Autodesk Fusion 360 part; units mm, degrees
(part 2 of 7)
  spline S15 degree 5 poles (6.7493, -2.5075) (6.7469, -2.5043) (6.7422, -2.4978) (6.7351, -2.4882) (6.7256, -2.4755) (6.7136, -2.4596) (6.7016, -2.4438) (6.6895, -2.4282) (6.6774, -2.4126) (6.6652, -2.3971) (6.653, -2.3817) (6.6407, -2.3664) (6.6283, -2.3512) (6.6159, -2.336) (6.6034, -2.321) (6.5909, -2.3061) (6.5783, -2.2913) (6.5657, -2.2766) (6.553, -2.2619) (6.5402, -2.2474) (6.5274, -2.233) (6.5145, -2.2186) (6.5016, -2.2044) (6.4886, -2.1903) (6.4756, -2.1763) (6.4625, -2.1624) (6.4493, -2.1486) (6.4361, -2.1349) (6.4229, -2.1213) (6.4095, -2.1078) (6.3962, -2.0944) (6.3827, -2.0812) (6.3692, -2.068) (6.3557, -2.055) (6.3421, -2.0421) (6.3284, -2.0293) (6.3147, -2.0166) (6.301, -2.004) (6.2871, -1.9916) (6.2733, -1.9792) (6.2593, -1.967) (6.2453, -1.955) (6.2313, -1.943) (6.2172, -1.9312) (6.203, -1.9195) (6.1888, -1.9079) (6.1745, -1.8965) (6.1602, -1.8852) (6.1458, -1.874) (6.1313, -1.863) (6.1168, -1.8521) (6.1023, -1.8414) (6.0876, -1.8308) (6.0729, -1.8204) (6.0582, -1.8101) (6.0434, -1.8) (6.0285, -1.79) (6.0136, -1.7802) (5.9986, -1.7705) (5.9836, -1.761) (5.9685, -1.7518) (5.9533, -1.7427) (5.938, -1.7339) (5.9226, -1.7254) (5.9071, -1.717) (5.8916, -1.7089) (5.8761, -1.7008) (5.8605, -1.6929) (5.8448, -1.6852) (5.8291, -1.6778) (5.8132, -1.671) (5.8002, -1.6661) (5.7904, -1.6628) (5.7838, -1.6608) (5.7805, -1.6598) knots -1 -1 -1 -1 -1 -1 -0.98571429 -0.97142857 -0.95714286 -0.94285714 -0.92857143 -0.91428571 -0.9 -0.88571429 -0.87142857 -0.85714286 -0.84285714 -0.82857143 -0.81428571 -0.8 -0.78571429 -0.77142857 -0.75714286 -0.74285714 -0.72857143 -0.71428571 -0.7 -0.68571429 -0.67142857 -0.65714286 -0.64285714 -0.62857143 -0.61428571 -0.6 -0.58571429 -0.57142857 -0.55714286 -0.54285714 -0.52857143 -0.51428571 -0.5 -0.48571429 -0.47142857 -0.45714286 -0.44285714 -0.42857143 -0.41428571 -0.4 -0.38571429 -0.37142857 -0.35714286 -0.34285714 -0.32857143 -0.31428571 -0.3 -0.28571429 -0.27142857 -0.25714286 -0.24285714 -0.22857143 -0.21428571 -0.2 -0.18571429 -0.17142857 -0.15714286 -0.14285714 -0.12857143 -0.11428571 -0.1 -0.08571429 -0.07142857 -0.05714286 -0.04285714 -0.02857143 -0.01428571 0 0 0 0 0 0
  line L15 (5.7805, -1.6598) -> (5.4506, -1.5651)
  arc A31 (5.3118, -1.3245) -> (5.4506, -1.5651) centre (5.5058, -1.3729) ccw
  arc A32 (5.3118, -1.3245) -> (5.4143, -0.8091) centre (0, 0) ccw
  arc A33 (5.6347, -0.6399) -> (5.4143, -0.8091) centre (5.6121, -0.8386) ccw
  line L16 (5.6347, -0.6399) -> (5.9756, -0.6786)
  spline S16 degree 5 poles (5.9756, -0.6786) (5.9791, -0.679) (5.9859, -0.6797) (5.9963, -0.6804) (6.0101, -0.6808) (6.0275, -0.6806) (6.0448, -0.6798) (6.0622, -0.6786) (6.0796, -0.6773) (6.0971, -0.6758) (6.1145, -0.6742) (6.132, -0.6724) (6.1495, -0.6704) (6.167, -0.6682) (6.1845, -0.6656) (6.202, -0.6628) (6.2196, -0.6598) (6.2371, -0.6566) (6.2546, -0.6532) (6.2722, -0.6497) (6.2897, -0.646) (6.3073, -0.6422) (6.3249, -0.6382) (6.3424, -0.634) (6.36, -0.6297) (6.3776, -0.6252) (6.3951, -0.6205) (6.4127, -0.6157) (6.4303, -0.6108) (6.4478, -0.6057) (6.4654, -0.6004) (6.4829, -0.595) (6.5005, -0.5895) (6.5181, -0.5838) (6.5356, -0.578) (6.5532, -0.5721) (6.5707, -0.566) (6.5882, -0.5598) (6.6058, -0.5535) (6.6233, -0.547) (6.6408, -0.5404) (6.6583, -0.5336) (6.6758, -0.5268) (6.6933, -0.5198) (6.7108, -0.5127) (6.7283, -0.5055) (6.7457, -0.4981) (6.7632, -0.4906) (6.7806, -0.483) (6.7981, -0.4753) (6.8155, -0.4675) (6.8329, -0.4595) (6.8503, -0.4514) (6.8677, -0.4432) (6.8851, -0.4349) (6.9024, -0.4265) (6.9198, -0.418) (6.9371, -0.4093) (6.9544, -0.4006) (6.9717, -0.3917) (6.989, -0.3827) (7.0063, -0.3736) (7.0235, -0.3644) (7.0408, -0.355) (7.058, -0.3456) (7.0752, -0.3361) (7.0924, -0.3264) (7.1095, -0.3167) (7.1267, -0.3068) (7.1438, -0.2968) (7.1609, -0.2867) (7.1746, -0.2786) (7.1848, -0.2724) (7.1917, -0.2683) (7.1951, -0.2662) knots 0 0 0 0 0 0 0.01428571 0.02857143 0.04285714 0.05714286 0.07142857 0.08571429 0.1 0.11428571 0.12857143 0.14285714 0.15714286 0.17142857 0.18571429 0.2 0.21428571 0.22857143 0.24285714 0.25714286 0.27142857 0.28571429 0.3 0.31428571 0.32857143 0.34285714 0.35714286 0.37142857 0.38571429 0.4 0.41428571 0.42857143 0.44285714 0.45714286 0.47142857 0.48571429 0.5 0.51428571 0.52857143 0.54285714 0.55714286 0.57142857 0.58571429 0.6 0.61428571 0.62857143 0.64285714 0.65714286 0.67142857 0.68571429 0.7 0.71428571 0.72857143 0.74285714 0.75714286 0.77142857 0.78571429 0.8 0.81428571 0.82857143 0.84285714 0.85714286 0.87142857 0.88571429 0.9 0.91428571 0.92857143 0.94285714 0.95714286 0.97142857 0.98571429 1 1 1 1 1 1
  arc A34 (7.1951, -0.2662) -> (7.1951, 0.2662) centre (0, 0) ccw
  spline S17 degree 5 poles (7.1951, 0.2662) (7.1917, 0.2683) (7.1848, 0.2724) (7.1746, 0.2786) (7.1609, 0.2867) (7.1438, 0.2968) (7.1267, 0.3068) (7.1095, 0.3167) (7.0924, 0.3264) (7.0752, 0.3361) (7.058, 0.3456) (7.0408, 0.355) (7.0235, 0.3644) (7.0063, 0.3736) (6.989, 0.3827) (6.9717, 0.3917) (6.9544, 0.4006) (6.9371, 0.4093) (6.9198, 0.418) (6.9024, 0.4265) (6.8851, 0.4349) (6.8677, 0.4432) (6.8503, 0.4514) (6.8329, 0.4595) (6.8155, 0.4675) (6.7981, 0.4753) (6.7806, 0.483) (6.7632, 0.4906) (6.7457, 0.4981) (6.7283, 0.5055) (6.7108, 0.5127) (6.6933, 0.5198) (6.6758, 0.5268) (6.6583, 0.5336) (6.6408, 0.5404) (6.6233, 0.547) (6.6058, 0.5535) (6.5882, 0.5598) (6.5707, 0.566) (6.5532, 0.5721) (6.5356, 0.578) (6.5181, 0.5838) (6.5005, 0.5895) (6.4829, 0.595) (6.4654, 0.6004) (6.4478, 0.6057) (6.4303, 0.6108) (6.4127, 0.6157) (6.3951, 0.6205) (6.3776, 0.6252) (6.36, 0.6297) (6.3424, 0.634) (6.3249, 0.6382) (6.3073, 0.6422) (6.2897, 0.646) (6.2722, 0.6497) (6.2546, 0.6532) (6.2371, 0.6566) (6.2196, 0.6598) (6.202, 0.6628) (6.1845, 0.6656) (6.167, 0.6682) (6.1495, 0.6704) (6.132, 0.6724) (6.1145, 0.6742) (6.0971, 0.6758) (6.0796, 0.6773) (6.0622, 0.6786) (6.0448, 0.6798) (6.0275, 0.6806) (6.0101, 0.6808) (5.9963, 0.6804) (5.9859, 0.6797) (5.9791, 0.679) (5.9756, 0.6786) knots -1 -1 -1 -1 -1 -1 -0.98571429 -0.97142857 -0.95714286 -0.94285714 -0.92857143 -0.91428571 -0.9 -0.88571429 -0.87142857 -0.85714286 -0.84285714 -0.82857143 -0.81428571 -0.8 -0.78571429 -0.77142857 -0.75714286 -0.74285714 -0.72857143 -0.71428571 -0.7 -0.68571429 -0.67142857 -0.65714286 -0.64285714 -0.62857143 -0.61428571 -0.6 -0.58571429 -0.57142857 -0.55714286 -0.54285714 -0.52857143 -0.51428571 -0.5 -0.48571429 -0.47142857 -0.45714286 -0.44285714 -0.42857143 -0.41428571 -0.4 -0.38571429 -0.37142857 -0.35714286 -0.34285714 -0.32857143 -0.31428571 -0.3 -0.28571429 -0.27142857 -0.25714286 -0.24285714 -0.22857143 -0.21428571 -0.2 -0.18571429 -0.17142857 -0.15714286 -0.14285714 -0.12857143 -0.11428571 -0.1 -0.08571429 -0.07142857 -0.05714286 -0.04285714 -0.02857143 -0.01428571 0 0 0 0 0 0
  line L17 (5.9756, 0.6786) -> (5.6347, 0.6399)
  arc A35 (5.4143, 0.8091) -> (5.6347, 0.6399) centre (5.6121, 0.8386) ccw
  arc A36 (5.4143, 0.8091) -> (5.3118, 1.3245) centre (0, 0) ccw
  arc A37 (5.4506, 1.5651) -> (5.3118, 1.3245) centre (5.5058, 1.3729) ccw
  line L18 (5.4506, 1.5651) -> (5.7805, 1.6598)
  spline S18 degree 5 poles (5.7805, 1.6598) (5.7838, 1.6608) (5.7904, 1.6628) (5.8002, 1.6661) (5.8132, 1.671) (5.8291, 1.6778) (5.8448, 1.6852) (5.8605, 1.6929) (5.8761, 1.7008) (5.8916, 1.7089) (5.9071, 1.717) (5.9226, 1.7254) (5.938, 1.7339) (5.9533, 1.7427) (5.9685, 1.7518) (5.9836, 1.761) (5.9986, 1.7705) (6.0136, 1.7802) (6.0285, 1.79) (6.0434, 1.8) (6.0582, 1.8101) (6.0729, 1.8204) (6.0876, 1.8308) (6.1023, 1.8414) (6.1168, 1.8521) (6.1313, 1.863) (6.1458, 1.874) (6.1602, 1.8852) (6.1745, 1.8965) (6.1888, 1.9079) (6.203, 1.9195) (6.2172, 1.9312) (6.2313, 1.943) (6.2453, 1.955) (6.2593, 1.967) (6.2733, 1.9792) (6.2871, 1.9916) (6.301, 2.004) (6.3147, 2.0166) (6.3284, 2.0293) (6.3421, 2.0421) (6.3557, 2.055) (6.3692, 2.068) (6.3827, 2.0812) (6.3962, 2.0944) (6.4095, 2.1078) (6.4229, 2.1213) (6.4361, 2.1349) (6.4493, 2.1486) (6.4625, 2.1624) (6.4756, 2.1763) (6.4886, 2.1903) (6.5016, 2.2044) (6.5145, 2.2186) (6.5274, 2.233) (6.5402, 2.2474) (6.553, 2.2619) (6.5657, 2.2766) (6.5783, 2.2913) (6.5909, 2.3061) (6.6034, 2.321) (6.6159, 2.336) (6.6283, 2.3512) (6.6407, 2.3664) (6.653, 2.3817) (6.6652, 2.3971) (6.6774, 2.4126) (6.6895, 2.4282) (6.7016, 2.4438) (6.7136, 2.4596) (6.7256, 2.4755) (6.7351, 2.4882) (6.7422, 2.4978) (6.7469, 2.5043) (6.7493, 2.5075) knots 0 0 0 0 0 0 0.01428571 0.02857143 0.04285714 0.05714286 0.07142857 0.08571429 0.1 0.11428571 0.12857143 0.14285714 0.15714286 0.17142857 0.18571429 0.2 0.21428571 0.22857143 0.24285714 0.25714286 0.27142857 0.28571429 0.3 0.31428571 0.32857143 0.34285714 0.35714286 0.37142857 0.38571429 0.4 0.41428571 0.42857143 0.44285714 0.45714286 0.47142857 0.48571429 0.5 0.51428571 0.52857143 0.54285714 0.55714286 0.57142857 0.58571429 0.6 0.61428571 0.62857143 0.64285714 0.65714286 0.67142857 0.68571429 0.7 0.71428571 0.72857143 0.74285714 0.75714286 0.77142857 0.78571429 0.8 0.81428571 0.82857143 0.84285714 0.85714286 0.87142857 0.88571429 0.9 0.91428571 0.92857143 0.94285714 0.95714286 0.97142857 0.98571429 1 1 1 1 1 1
  arc A38 (6.7493, 2.5075) -> (6.5455, 2.9994) centre (0, 0) ccw
  spline S19 degree 5 poles (6.5455, 2.9994) (6.5416, 3) (6.5337, 3.0012) (6.5219, 3.003) (6.5061, 3.0053) (6.4864, 3.008) (6.4668, 3.0107) (6.4472, 3.0133) (6.4276, 3.0157) (6.408, 3.018) (6.3885, 3.0203) (6.3689, 3.0224) (6.3495, 3.0244) (6.33, 3.0263) (6.3105, 3.0281) (6.2911, 3.0298) (6.2718, 3.0314) (6.2524, 3.0329) (6.2331, 3.0342) (6.2138, 3.0355) (6.1945, 3.0366) (6.1753, 3.0377) (6.1561, 3.0386) (6.1369, 3.0394) (6.1178, 3.0401) (6.0987, 3.0406) (6.0796, 3.0411) (6.0606, 3.0414) (6.0416, 3.0417) (6.0227, 3.0418) (6.0038, 3.0418) (5.9849, 3.0417) (5.9661, 3.0414) (5.9473, 3.0411) (5.9285, 3.0406) (5.9098, 3.04) (5.8911, 3.0392) (5.8725, 3.0384) (5.8539, 3.0374) (5.8354, 3.0363) (5.8169, 3.0351) (5.7985, 3.0338) (5.7801, 3.0323) (5.7618, 3.0307) (5.7435, 3.0289) (5.7252, 3.027) (5.7071, 3.025) (5.6889, 3.0229) (5.6709, 3.0206) (5.6528, 3.0182) (5.6349, 3.0156) (5.617, 3.0129) (5.5992, 3.0101) (5.5814, 3.007) (5.5637, 3.0038) (5.5461, 3.0005) (5.5286, 2.997) (5.5111, 2.9934) (5.4936, 2.9897) (5.4763, 2.9858) (5.459, 2.9817) (5.4419, 2.9773) (5.4248, 2.9727) (5.4079, 2.9679) (5.3911, 2.9628) (5.3744, 2.9576) (5.3577, 2.9523) (5.3411, 2.9469) (5.3245, 2.9413) (5.3082, 2.9354) (5.2921, 2.929) (5.2795, 2.9233) (5.2702, 2.9187) (5.2641, 2.9154) (5.2611, 2.9137) knots -1 -1 -1 -1 -1 -1 -0.98571429 -0.97142857 -0.95714286 -0.94285714 -0.92857143 -0.91428571 -0.9 -0.88571429 -0.87142857 -0.85714286 -0.84285714 -0.82857143 -0.81428571 -0.8 -0.78571429 -0.77142857 -0.75714286 -0.74285714 -0.72857143 -0.71428571 -0.7 -0.68571429 -0.67142857 -0.65714286 -0.64285714 -0.62857143 -0.61428571 -0.6 -0.58571429 -0.57142857 -0.55714286 -0.54285714 -0.52857143 -0.51428571 -0.5 -0.48571429 -0.47142857 -0.45714286 -0.44285714 -0.42857143 -0.41428571 -0.4 -0.38571429 -0.37142857 -0.35714286 -0.34285714 -0.32857143 -0.31428571 -0.3 -0.28571429 -0.27142857 -0.25714286 -0.24285714 -0.22857143 -0.21428571 -0.2 -0.18571429 -0.17142857 -0.15714286 -0.14285714 -0.12857143 -0.11428571 -0.1 -0.08571429 -0.07142857 -0.05714286 -0.04285714 -0.02857143 -0.01428571 0 0 0 0 0 0
  line L19 (5.2611, 2.9137) -> (4.9609, 2.7475)
  arc A39 (4.6925, 2.8194) -> (4.9609, 2.7475) centre (4.864, 2.9224) ccw
  arc A40 (4.6925, 2.8194) -> (4.4006, 3.2564) centre (0, 0) ccw
  arc A41 (4.4368, 3.5318) -> (4.4006, 3.2564) centre (4.5613, 3.3754) ccw
  line L20 (4.4368, 3.5318) -> (4.7053, 3.7456)
  spline S20 degree 5 poles (4.7053, 3.7456) (4.708, 3.7477) (4.7133, 3.7521) (4.7211, 3.7589) (4.7312, 3.7684) (4.7433, 3.7808) (4.755, 3.7937) (4.7665, 3.8068) (4.7779, 3.82) (4.7892, 3.8334) (4.8004, 3.8469) (4.8115, 3.8605) (4.8224, 3.8743) (4.8332, 3.8883) (4.8438, 3.9024) (4.8542, 3.9168) (4.8644, 3.9313) (4.8746, 3.946) (4.8846, 3.9608) (4.8945, 3.9757) (4.9043, 3.9907) (4.914, 4.0058) (4.9236, 4.0211) (4.9331, 4.0364) (4.9425, 4.0519) (4.9517, 4.0675) (4.9608, 4.0832) (4.9698, 4.0991) (4.9788, 4.115) (4.9876, 4.131) (4.9963, 4.1472) (5.0049, 4.1634) (5.0134, 4.1797) (5.0218, 4.1961) (5.0301, 4.2126) (5.0383, 4.2293) (5.0464, 4.246) (5.0544, 4.2628) (5.0623, 4.2796) (5.0701, 4.2966) (5.0779, 4.3137) (5.0855, 4.3308) (5.093, 4.348) (5.1004, 4.3653) (5.1078, 4.3827) (5.115, 4.4002) (5.1222, 4.4177) (5.1292, 4.4354) (5.1362, 4.4531) (5.1431, 4.4709) (5.1498, 4.4887) (5.1565, 4.5067) (5.1631, 4.5247) (5.1696, 4.5428) (5.176, 4.5609) (5.1823, 4.5792) (5.1886, 4.5975) (5.1947, 4.6158) (5.2007, 4.6343) (5.2067, 4.6528) (5.2126, 4.6714) (5.2183, 4.69) (5.224, 4.7087) (5.2296, 4.7275) (5.2351, 4.7464) (5.2405, 4.7653) (5.2459, 4.7843) (5.2511, 4.8033) (5.2563, 4.8224) (5.2613, 4.8416) (5.2663, 4.8608) (5.2702, 4.8762) (5.2731, 4.8878) (5.275, 4.8956) (5.2759, 4.8994) knots 0 0 0 0 0 0 0.01428571 0.02857143 0.04285714 0.05714286 0.07142857 0.08571429 0.1 0.11428571 0.12857143 0.14285714 0.15714286 0.17142857 0.18571429 0.2 0.21428571 0.22857143 0.24285714 0.25714286 0.27142857 0.28571429 0.3 0.31428571 0.32857143 0.34285714 0.35714286 0.37142857 0.38571429 0.4 0.41428571 0.42857143 0.44285714 0.45714286 0.47142857 0.48571429 0.5 0.51428571 0.52857143 0.54285714 0.55714286 0.57142857 0.58571429 0.6 0.61428571 0.62857143 0.64285714 0.65714286 0.67142857 0.68571429 0.7 0.71428571 0.72857143 0.74285714 0.75714286 0.77142857 0.78571429 0.8 0.81428571 0.82857143 0.84285714 0.85714286 0.87142857 0.88571429 0.9 0.91428571 0.92857143 0.94285714 0.95714286 0.97142857 0.98571429 1 1 1 1 1 1
  arc A42 (5.2759, 4.8994) -> (4.8994, 5.2759) centre (0, 0) ccw
  spline S21 degree 5 poles (4.8994, 5.2759) (4.8956, 5.275) (4.8878, 5.2731) (4.8762, 5.2702) (4.8608, 5.2663) (4.8416, 5.2613) (4.8224, 5.2563) (4.8033, 5.2511) (4.7843, 5.2459) (4.7653, 5.2405) (4.7464, 5.2351) (4.7275, 5.2296) (4.7087, 5.224) (4.69, 5.2183) (4.6714, 5.2126) (4.6528, 5.2067) (4.6343, 5.2007) (4.6158, 5.1947) (4.5975, 5.1886) (4.5792, 5.1823) (4.5609, 5.176) (4.5428, 5.1696) (4.5247, 5.1631) (4.5067, 5.1565) (4.4887, 5.1498) (4.4709, 5.1431) (4.4531, 5.1362) (4.4354, 5.1292) (4.4177, 5.1222) (4.4002, 5.115) (4.3827, 5.1078) (4.3653, 5.1004) (4.348, 5.093) (4.3308, 5.0855) (4.3137, 5.0779) (4.2966, 5.0701) (4.2796, 5.0623) (4.2628, 5.0544) (4.246, 5.0464) (4.2293, 5.0383) (4.2126, 5.0301) (4.1961, 5.0218) (4.1797, 5.0134) (4.1634, 5.0049) (4.1472, 4.9963) (4.131, 4.9876) (4.115, 4.9788) (4.0991, 4.9698) (4.0832, 4.9608) (4.0675, 4.9517) (4.0519, 4.9425) (4.0364, 4.9331) (4.0211, 4.9236) (4.0058, 4.914) (3.9907, 4.9043) (3.9757, 4.8945) (3.9608, 4.8846) (3.946, 4.8746) (3.9313, 4.8644) (3.9168, 4.8542) (3.9024, 4.8438) (3.8883, 4.8332) (3.8743, 4.8224) (3.8605, 4.8115) (3.8469, 4.8004) (3.8334, 4.7892) (3.82, 4.7779) (3.8068, 4.7665) (3.7937, 4.755) (3.7808, 4.7433) (3.7684, 4.7312) (3.7589, 4.7211) (3.7521, 4.7133) (3.7477, 4.708) (3.7456, 4.7053) knots -1 -1 -1 -1 -1 -1 -0.98571429 -0.97142857 -0.95714286 -0.94285714 -0.92857143 -0.91428571 -0.9 -0.88571429 -0.87142857 -0.85714286 -0.84285714 -0.82857143 -0.81428571 -0.8 -0.78571429 -0.77142857 -0.75714286 -0.74285714 -0.72857143 -0.71428571 -0.7 -0.68571429 -0.67142857 -0.65714286 -0.64285714 -0.62857143 -0.61428571 -0.6 -0.58571429 -0.57142857 -0.55714286 -0.54285714 -0.52857143 -0.51428571 -0.5 -0.48571429 -0.47142857 -0.45714286 -0.44285714 -0.42857143 -0.41428571 -0.4 -0.38571429 -0.37142857 -0.35714286 -0.34285714 -0.32857143 -0.31428571 -0.3 -0.28571429 -0.27142857 -0.25714286 -0.24285714 -0.22857143 -0.21428571 -0.2 -0.18571429 -0.17142857 -0.15714286 -0.14285714 -0.12857143 -0.11428571 -0.1 -0.08571429 -0.07142857 -0.05714286 -0.04285714 -0.02857143 -0.01428571 0 0 0 0 0 0
  line L21 (3.7456, 4.7053) -> (3.5318, 4.4368)
  arc A43 (3.2564, 4.4006) -> (3.5318, 4.4368) centre (3.3754, 4.5613) ccw
  arc A44 (3.2564, 4.4006) -> (2.8194, 4.6925) centre (0, 0) ccw
  arc A45 (2.7475, 4.9609) -> (2.8194, 4.6925) centre (2.9224, 4.864) ccw
  line L22 (2.7475, 4.9609) -> (2.9137, 5.2611)
  spline S22 degree 5 poles (2.9137, 5.2611) (2.9154, 5.2641) (2.9187, 5.2702) (2.9233, 5.2795) (2.929, 5.2921) (2.9354, 5.3082) (2.9413, 5.3245) (2.9469, 5.3411) (2.9523, 5.3577) (2.9576, 5.3744) (2.9628, 5.3911) (2.9679, 5.4079) (2.9727, 5.4248) (2.9773, 5.4419) (2.9817, 5.459) (2.9858, 5.4763) (2.9897, 5.4936) (2.9934, 5.5111) (2.997, 5.5286) (3.0005, 5.5461) (3.0038, 5.5637) (3.007, 5.5814) (3.0101, 5.5992) (3.0129, 5.617) (3.0156, 5.6349) (3.0182, 5.6528) (3.0206, 5.6709) (3.0229, 5.6889) (3.025, 5.7071) (3.027, 5.7252) (3.0289, 5.7435) (3.0307, 5.7618) (3.0323, 5.7801) (3.0338, 5.7985) (3.0351, 5.8169) (3.0363, 5.8354) (3.0374, 5.8539) (3.0384, 5.8725) (3.0392, 5.8911) (3.04, 5.9098) (3.0406, 5.9285) (3.0411, 5.9473) (3.0414, 5.9661) (3.0417, 5.9849) (3.0418, 6.0038) (3.0418, 6.0227) (3.0417, 6.0416) (3.0414, 6.0606) (3.0411, 6.0796) (3.0406, 6.0987) (3.0401, 6.1178) (3.0394, 6.1369) (3.0386, 6.1561) (3.0377, 6.1753) (3.0366, 6.1945) (3.0355, 6.2138) (3.0342, 6.2331) (3.0329, 6.2524) (3.0314, 6.2718) (3.0298, 6.2911) (3.0281, 6.3105) (3.0263, 6.33) (3.0244, 6.3495) (3.0224, 6.3689) (3.0203, 6.3885) (3.018, 6.408) (3.0157, 6.4276) (3.0133, 6.4472) (3.0107, 6.4668) (3.008, 6.4864) (3.0053, 6.5061) (3.003, 6.5219) (3.0012, 6.5337) (3, 6.5416) (2.9994, 6.5455) knots 0 0 0 0 0 0 0.01428571 0.02857143 0.04285714 0.05714286 0.07142857 0.08571429 0.1 0.11428571 0.12857143 0.14285714 0.15714286 0.17142857 0.18571429 0.2 0.21428571 0.22857143 0.24285714 0.25714286 0.27142857 0.28571429 0.3 0.31428571 0.32857143 0.34285714 0.35714286 0.37142857 0.38571429 0.4 0.41428571 0.42857143 0.44285714 0.45714286 0.47142857 0.48571429 0.5 0.51428571 0.52857143 0.54285714 0.55714286 0.57142857 0.58571429 0.6 0.61428571 0.62857143 0.64285714 0.65714286 0.67142857 0.68571429 0.7 0.71428571 0.72857143 0.74285714 0.75714286 0.77142857 0.78571429 0.8 0.81428571 0.82857143 0.84285714 0.85714286 0.87142857 0.88571429 0.9 0.91428571 0.92857143 0.94285714 0.95714286 0.97142857 0.98571429 1 1 1 1 1 1
  arc A46 (2.9994, 6.5455) -> (2.5075, 6.7493) centre (0, 0) ccw
  spline S23 degree 5 poles (2.5075, 6.7493) (2.5043, 6.7469) (2.4978, 6.7422) (2.4882, 6.7351) (2.4755, 6.7256) (2.4596, 6.7136) (2.4438, 6.7016) (2.4282, 6.6895) (2.4126, 6.6774) (2.3971, 6.6652) (2.3817, 6.653) (2.3664, 6.6407) (2.3512, 6.6283) (2.336, 6.6159) (2.321, 6.6034) (2.3061, 6.5909) (2.2913, 6.5783) (2.2766, 6.5657) (2.2619, 6.553) (2.2474, 6.5402) (2.233, 6.5274) (2.2186, 6.5145) (2.2044, 6.5016) (2.1903, 6.4886) (2.1763, 6.4756) (2.1624, 6.4625) (2.1486, 6.4493) (2.1349, 6.4361) (2.1213, 6.4229) (2.1078, 6.4095) (2.0944, 6.3962) (2.0812, 6.3827) (2.068, 6.3692) (2.055, 6.3557) (2.0421, 6.3421) (2.0293, 6.3284) (2.0166, 6.3147) (2.004, 6.301) (1.9916, 6.2871) (1.9792, 6.2733) (1.967, 6.2593) (1.955, 6.2453) (1.943, 6.2313) (1.9312, 6.2172) (1.9195, 6.203) (1.9079, 6.1888) (1.8965, 6.1745) (1.8852, 6.1602) (1.874, 6.1458) (1.863, 6.1313) (1.8521, 6.1168) (1.8414, 6.1023) (1.8308, 6.0876) (1.8204, 6.0729) (1.8101, 6.0582) (1.8, 6.0434) (1.79, 6.0285) (1.7802, 6.0136) (1.7705, 5.9986) (1.761, 5.9836) (1.7518, 5.9685) (1.7427, 5.9533) (1.7339, 5.938) (1.7254, 5.9226) (1.717, 5.9071) (1.7089, 5.8916) (1.7008, 5.8761) (1.6929, 5.8605) (1.6852, 5.8448) (1.6778, 5.8291) (1.671, 5.8132) (1.6661, 5.8002) (1.6628, 5.7904) (1.6608, 5.7838) (1.6598, 5.7805) knots -1 -1 -1 -1 -1 -1 -0.98571429 -0.97142857 -0.95714286 -0.94285714 -0.92857143 -0.91428571 -0.9 -0.88571429 -0.87142857 -0.85714286 -0.84285714 -0.82857143 -0.81428571 -0.8 -0.78571429 -0.77142857 -0.75714286 -0.74285714 -0.72857143 -0.71428571 -0.7 -0.68571429 -0.67142857 -0.65714286 -0.64285714 -0.62857143 -0.61428571 -0.6 -0.58571429 -0.57142857 -0.55714286 -0.54285714 -0.52857143 -0.51428571 -0.5 -0.48571429 -0.47142857 -0.45714286 -0.44285714 -0.42857143 -0.41428571 -0.4 -0.38571429 -0.37142857 -0.35714286 -0.34285714 -0.32857143 -0.31428571 -0.3 -0.28571429 -0.27142857 -0.25714286 -0.24285714 -0.22857143 -0.21428571 -0.2 -0.18571429 -0.17142857 -0.15714286 -0.14285714 -0.12857143 -0.11428571 -0.1 -0.08571429 -0.07142857 -0.05714286 -0.04285714 -0.02857143 -0.01428571 0 0 0 0 0 0
  line L23 (1.6598, 5.7805) -> (1.5651, 5.4506)
  arc A47 (1.3245, 5.3118) -> (1.5651, 5.4506) centre (1.3729, 5.5058) ccw
  arc A48 (1.3245, 5.3118) -> (0.8091, 5.4143) centre (0, 0) ccw
  arc A49 (0.6399, 5.6347) -> (0.8091, 5.4143) centre (0.8386, 5.6121) ccw
  line L24 (0.6399, 5.6347) -> (0.6786, 5.9756)
  spline S24 degree 5 poles (0.6786, 5.9756) (0.679, 5.9791) (0.6797, 5.9859) (0.6804, 5.9963) (0.6808, 6.0101) (0.6806, 6.0275) (0.6798, 6.0448) (0.6786, 6.0622) (0.6773, 6.0796) (0.6758, 6.0971) (0.6742, 6.1145) (0.6724, 6.132) (0.6704, 6.1495) (0.6682, 6.167) (0.6656, 6.1845) (0.6628, 6.202) (0.6598, 6.2196) (0.6566, 6.2371) (0.6532, 6.2546) (0.6497, 6.2722) (0.646, 6.2897) (0.6422, 6.3073) (0.6382, 6.3249) (0.634, 6.3424) (0.6297, 6.36) (0.6252, 6.3776) (0.6205, 6.3951) (0.6157, 6.4127) (0.6108, 6.4303) (0.6057, 6.4478) (0.6004, 6.4654) (0.595, 6.4829) (0.5895, 6.5005) (0.5838, 6.5181) (0.578, 6.5356) (0.5721, 6.5532) (0.566, 6.5707) (0.5598, 6.5882) (0.5535, 6.6058) (0.547, 6.6233) (0.5404, 6.6408) (0.5336, 6.6583) (0.5268, 6.6758) (0.5198, 6.6933) (0.5127, 6.7108) (0.5055, 6.7283) (0.4981, 6.7457) (0.4906, 6.7632) (0.483, 6.7806) (0.4753, 6.7981) (0.4675, 6.8155) (0.4595, 6.8329) (0.4514, 6.8503) (0.4432, 6.8677) (0.4349, 6.8851) (0.4265, 6.9024) (0.418, 6.9198) (0.4093, 6.9371) (0.4006, 6.9544) (0.3917, 6.9717) (0.3827, 6.989) (0.3736, 7.0063) (0.3644, 7.0235) (0.355, 7.0408) (0.3456, 7.058) (0.3361, 7.0752) (0.3264, 7.0924) (0.3167, 7.1095) (0.3068, 7.1267) (0.2968, 7.1438) (0.2867, 7.1609) (0.2786, 7.1746) (0.2724, 7.1848) (0.2683, 7.1917) (0.2662, 7.1951) knots 0 0 0 0 0 0 0.01428571 0.02857143 0.04285714 0.05714286 0.07142857 0.08571429 0.1 0.11428571 0.12857143 0.14285714 0.15714286 0.17142857 0.18571429 0.2 0.21428571 0.22857143 0.24285714 0.25714286 0.27142857 0.28571429 0.3 0.31428571 0.32857143 0.34285714 0.35714286 0.37142857 0.38571429 0.4 0.41428571 0.42857143 0.44285714 0.45714286 0.47142857 0.48571429 0.5 0.51428571 0.52857143 0.54285714 0.55714286 0.57142857 0.58571429 0.6 0.61428571 0.62857143 0.64285714 0.65714286 0.67142857 0.68571429 0.7 0.71428571 0.72857143 0.74285714 0.75714286 0.77142857 0.78571429 0.8 0.81428571 0.82857143 0.84285714 0.85714286 0.87142857 0.88571429 0.9 0.91428571 0.92857143 0.94285714 0.95714286 0.97142857 0.98571429 1 1 1 1 1 1
  arc A50 (0.2662, 7.1951) -> (-0.2662, 7.1951) centre (0, 0) ccw
  spline S25 degree 5 poles (-0.2662, 7.1951) (-0.2683, 7.1917) (-0.2724, 7.1848) (-0.2786, 7.1746) (-0.2867, 7.1609) (-0.2968, 7.1438) (-0.3068, 7.1267) (-0.3167, 7.1095) (-0.3264, 7.0924) (-0.3361, 7.0752) (-0.3456, 7.058) (-0.355, 7.0408) (-0.3644, 7.0235) (-0.3736, 7.0063) (-0.3827, 6.989) (-0.3917, 6.9717) (-0.4006, 6.9544) (-0.4093, 6.9371) (-0.418, 6.9198) (-0.4265, 6.9024) (-0.4349, 6.8851) (-0.4432, 6.8677) (-0.4514, 6.8503) (-0.4595, 6.8329) (-0.4675, 6.8155) (-0.4753, 6.7981) (-0.483, 6.7806) (-0.4906, 6.7632) (-0.4981, 6.7457) (-0.5055, 6.7283) (-0.5127, 6.7108) (-0.5198, 6.6933) (-0.5268, 6.6758) (-0.5336, 6.6583) (-0.5404, 6.6408) (-0.547, 6.6233) (-0.5535, 6.6058) (-0.5598, 6.5882) (-0.566, 6.5707) (-0.5721, 6.5532) (-0.578, 6.5356) (-0.5838, 6.5181) (-0.5895, 6.5005) (-0.595, 6.4829) (-0.6004, 6.4654) (-0.6057, 6.4478) (-0.6108, 6.4303) (-0.6157, 6.4127) (-0.6205, 6.3951) (-0.6252, 6.3776) (-0.6297, 6.36) (-0.634, 6.3424) (-0.6382, 6.3249) (-0.6422, 6.3073) (-0.646, 6.2897) (-0.6497, 6.2722) (-0.6532, 6.2546) (-0.6566, 6.2371) (-0.6598, 6.2196) (-0.6628, 6.202) (-0.6656, 6.1845) (-0.6682, 6.167) (-0.6704, 6.1495) (-0.6724, 6.132) (-0.6742, 6.1145) (-0.6758, 6.0971) (-0.6773, 6.0796) (-0.6786, 6.0622) (-0.6798, 6.0448) (-0.6806, 6.0275) (-0.6808, 6.0101) (-0.6804, 5.9963) (-0.6797, 5.9859) (-0.679, 5.9791) (-0.6786, 5.9756) knots -1 -1 -1 -1 -1 -1 -0.98571429 -0.97142857 -0.95714286 -0.94285714 -0.92857143 -0.91428571 -0.9 -0.88571429 -0.87142857 -0.85714286 -0.84285714 -0.82857143 -0.81428571 -0.8 -0.78571429 -0.77142857 -0.75714286 -0.74285714 -0.72857143 -0.71428571 -0.7 -0.68571429 -0.67142857 -0.65714286 -0.64285714 -0.62857143 -0.61428571 -0.6 -0.58571429 -0.57142857 -0.55714286 -0.54285714 -0.52857143 -0.51428571 -0.5 -0.48571429 -0.47142857 -0.45714286 -0.44285714 -0.42857143 -0.41428571 -0.4 -0.38571429 -0.37142857 -0.35714286 -0.34285714 -0.32857143 -0.31428571 -0.3 -0.28571429 -0.27142857 -0.25714286 -0.24285714 -0.22857143 -0.21428571 -0.2 -0.18571429 -0.17142857 -0.15714286 -0.14285714 -0.12857143 -0.11428571 -0.1 -0.08571429 -0.07142857 -0.05714286 -0.04285714 -0.02857143 -0.01428571 0 0 0 0 0 0
  line L25 (-0.6786, 5.9756) -> (-0.6399, 5.6347)
  arc A51 (-0.8091, 5.4143) -> (-0.6399, 5.6347) centre (-0.8386, 5.6121) ccw
  arc A52 (-0.8091, 5.4143) -> (-1.3245, 5.3118) centre (0, 0) ccw
  arc A53 (-1.5651, 5.4506) -> (-1.3245, 5.3118) centre (-1.3729, 5.5058) ccw
  line L26 (-1.5651, 5.4506) -> (-1.6598, 5.7805)
  spline S26 degree 5 poles (-1.6598, 5.7805) (-1.6608, 5.7838) (-1.6628, 5.7904) (-1.6661, 5.8002) (-1.671, 5.8132) (-1.6778, 5.8291) (-1.6852, 5.8448) (-1.6929, 5.8605) (-1.7008, 5.8761) (-1.7089, 5.8916) (-1.717, 5.9071) (-1.7254, 5.9226) (-1.7339, 5.938) (-1.7427, 5.9533) (-1.7518, 5.9685) (-1.761, 5.9836) (-1.7705, 5.9986) (-1.7802, 6.0136) (-1.79, 6.0285) (-1.8, 6.0434) (-1.8101, 6.0582) (-1.8204, 6.0729) (-1.8308, 6.0876) (-1.8414, 6.1023) (-1.8521, 6.1168) (-1.863, 6.1313) (-1.874, 6.1458) (-1.8852, 6.1602) (-1.8965, 6.1745) (-1.9079, 6.1888) (-1.9195, 6.203) (-1.9312, 6.2172) (-1.943, 6.2313) (-1.955, 6.2453) (-1.967, 6.2593) (-1.9792, 6.2733) (-1.9916, 6.2871) (-2.004, 6.301) (-2.0166, 6.3147) (-2.0293, 6.3284) (-2.0421, 6.3421) (-2.055, 6.3557) (-2.068, 6.3692) (-2.0812, 6.3827) (-2.0944, 6.3962) (-2.1078, 6.4095) (-2.1213, 6.4229) (-2.1349, 6.4361) (-2.1486, 6.4493) (-2.1624, 6.4625) (-2.1763, 6.4756) (-2.1903, 6.4886) (-2.2044, 6.5016) (-2.2186, 6.5145) (-2.233, 6.5274) (-2.2474, 6.5402) (-2.2619, 6.553) (-2.2766, 6.5657) (-2.2913, 6.5783) (-2.3061, 6.5909) (-2.321, 6.6034) (-2.336, 6.6159) (-2.3512, 6.6283) (-2.3664, 6.6407) (-2.3817, 6.653) (-2.3971, 6.6652) (-2.4126, 6.6774) (-2.4282, 6.6895) (-2.4438, 6.7016) (-2.4596, 6.7136) (-2.4755, 6.7256) (-2.4882, 6.7351) (-2.4978, 6.7422) (-2.5043, 6.7469) (-2.5075, 6.7493) knots 0 0 0 0 0 0 0.01428571 0.02857143 0.04285714 0.05714286 0.07142857 0.08571429 0.1 0.11428571 0.12857143 0.14285714 0.15714286 0.17142857 0.18571429 0.2 0.21428571 0.22857143 0.24285714 0.25714286 0.27142857 0.28571429 0.3 0.31428571 0.32857143 0.34285714 0.35714286 0.37142857 0.38571429 0.4 0.41428571 0.42857143 0.44285714 0.45714286 0.47142857 0.48571429 0.5 0.51428571 0.52857143 0.54285714 0.55714286 0.57142857 0.58571429 0.6 0.61428571 0.62857143 0.64285714 0.65714286 0.67142857 0.68571429 0.7 0.71428571 0.72857143 0.74285714 0.75714286 0.77142857 0.78571429 0.8 0.81428571 0.82857143 0.84285714 0.85714286 0.87142857 0.88571429 0.9 0.91428571 0.92857143 0.94285714 0.95714286 0.97142857 0.98571429 1 1 1 1 1 1
  arc A54 (-2.5075, 6.7493) -> (-2.9994, 6.5455) centre (0, 0) ccw
  spline S27 degree 5 poles (-2.9994, 6.5455) (-3, 6.5416) (-3.0012, 6.5337) (-3.003, 6.5219) (-3.0053, 6.5061) (-3.008, 6.4864) (-3.0107, 6.4668) (-3.0133, 6.4472) (-3.0157, 6.4276) (-3.018, 6.408) (-3.0203, 6.3885) (-3.0224, 6.3689) (-3.0244, 6.3495) (-3.0263, 6.33) (-3.0281, 6.3105) (-3.0298, 6.2911) (-3.0314, 6.2718) (-3.0329, 6.2524) (-3.0342, 6.2331) (-3.0355, 6.2138) (-3.0366, 6.1945) (-3.0377, 6.1753) (-3.0386, 6.1561) (-3.0394, 6.1369) (-3.0401, 6.1178) (-3.0406, 6.0987) (-3.0411, 6.0796) (-3.0414, 6.0606) (-3.0417, 6.0416) (-3.0418, 6.0227) (-3.0418, 6.0038) (-3.0417, 5.9849) (-3.0414, 5.9661) (-3.0411, 5.9473) (-3.0406, 5.9285) (-3.04, 5.9098) (-3.0392, 5.8911) (-3.0384, 5.8725) (-3.0374, 5.8539) (-3.0363, 5.8354) (-3.0351, 5.8169) (-3.0338, 5.7985) (-3.0323, 5.7801) (-3.0307, 5.7618) (-3.0289, 5.7435) (-3.027, 5.7252) (-3.025, 5.7071) (-3.0229, 5.6889) (-3.0206, 5.6709) (-3.0182, 5.6528) (-3.0156, 5.6349) (-3.0129, 5.617) (-3.0101, 5.5992) (-3.007, 5.5814) (-3.0038, 5.5637) (-3.0005, 5.5461) (-2.997, 5.5286) (-2.9934, 5.5111) (-2.9897, 5.4936) (-2.9858, 5.4763) (-2.9817, 5.459) (-2.9773, 5.4419) (-2.9727, 5.4248) (-2.9679, 5.4079) (-2.9628, 5.3911) (-2.9576, 5.3744) (-2.9523, 5.3577) (-2.9469, 5.3411) (-2.9413, 5.3245) (-2.9354, 5.3082) (-2.929, 5.2921) (-2.9233, 5.2795) (-2.9187, 5.2702) (-2.9154, 5.2641) (-2.9137, 5.2611) knots -1 -1 -1 -1 -1 -1 -0.98571429 -0.97142857 -0.95714286 -0.94285714 -0.92857143 -0.91428571 -0.9 -0.88571429 -0.87142857 -0.85714286 -0.84285714 -0.82857143 -0.81428571 -0.8 -0.78571429 -0.77142857 -0.75714286 -0.74285714 -0.72857143 -0.71428571 -0.7 -0.68571429 -0.67142857 -0.65714286 -0.64285714 -0.62857143 -0.61428571 -0.6 -0.58571429 -0.57142857 -0.55714286 -0.54285714 -0.52857143 -0.51428571 -0.5 -0.48571429 -0.47142857 -0.45714286 -0.44285714 -0.42857143 -0.41428571 -0.4 -0.38571429 -0.37142857 -0.35714286 -0.34285714 -0.32857143 -0.31428571 -0.3 -0.28571429 -0.27142857 -0.25714286 -0.24285714 -0.22857143 -0.21428571 -0.2 -0.18571429 -0.17142857 -0.15714286 -0.14285714 -0.12857143 -0.11428571 -0.1 -0.08571429 -0.07142857 -0.05714286 -0.04285714 -0.02857143 -0.01428571 0 0 0 0 0 0
  line L27 (-2.9137, 5.2611) -> (-2.7475, 4.9609)
  arc A55 (-2.8194, 4.6925) -> (-2.7475, 4.9609) centre (-2.9224, 4.864) ccw
  arc A56 (-2.8194, 4.6925) -> (-3.2564, 4.4006) centre (0, 0) ccw
  arc A57 (-3.5318, 4.4368) -> (-3.2564, 4.4006) centre (-3.3754, 4.5613) ccw
  line L28 (-3.5318, 4.4368) -> (-3.7456, 4.7053)
  spline S28 degree 5 poles (-3.7456, 4.7053) (-3.7477, 4.708) (-3.7521, 4.7133) (-3.7589, 4.7211) (-3.7684, 4.7312) (-3.7808, 4.7433) (-3.7937, 4.755) (-3.8068, 4.7665) (-3.82, 4.7779) (-3.8334, 4.7892) (-3.8469, 4.8004) (-3.8605, 4.8115) (-3.8743, 4.8224) (-3.8883, 4.8332) (-3.9024, 4.8438) (-3.9168, 4.8542) (-3.9313, 4.8644) (-3.946, 4.8746) (-3.9608, 4.8846) (-3.9757, 4.8945) (-3.9907, 4.9043) (-4.0058, 4.914) (-4.0211, 4.9236) (-4.0364, 4.9331) (-4.0519, 4.9425) (-4.0675, 4.9517) (-4.0832, 4.9608) (-4.0991, 4.9698) (-4.115, 4.9788) (-4.131, 4.9876) (-4.1472, 4.9963) (-4.1634, 5.0049) (-4.1797, 5.0134) (-4.1961, 5.0218) (-4.2126, 5.0301) (-4.2293, 5.0383) (-4.246, 5.0464) (-4.2628, 5.0544) (-4.2796, 5.0623) (-4.2966, 5.0701) (-4.3137, 5.0779) (-4.3308, 5.0855) (-4.348, 5.093) (-4.3653, 5.1004) (-4.3827, 5.1078) (-4.4002, 5.115) (-4.4177, 5.1222) (-4.4354, 5.1292) (-4.4531, 5.1362) (-4.4709, 5.1431) (-4.4887, 5.1498) (-4.5067, 5.1565) (-4.5247, 5.1631) (-4.5428, 5.1696) (-4.5609, 5.176) (-4.5792, 5.1823) (-4.5975, 5.1886) (-4.6158, 5.1947) (-4.6343, 5.2007) (-4.6528, 5.2067) (-4.6714, 5.2126) (-4.69, 5.2183) (-4.7087, 5.224) (-4.7275, 5.2296) (-4.7464, 5.2351) (-4.7653, 5.2405) (-4.7843, 5.2459) (-4.8033, 5.2511) (-4.8224, 5.2563) (-4.8416, 5.2613) (-4.8608, 5.2663) (-4.8762, 5.2702) (-4.8878, 5.2731) (-4.8956, 5.275) (-4.8994, 5.2759) knots 0 0 0 0 0 0 0.01428571 0.02857143 0.04285714 0.05714286 0.07142857 0.08571429 0.1 0.11428571 0.12857143 0.14285714 0.15714286 0.17142857 0.18571429 0.2 0.21428571 0.22857143 0.24285714 0.25714286 0.27142857 0.28571429 0.3 0.31428571 0.32857143 0.34285714 0.35714286 0.37142857 0.38571429 0.4 0.41428571 0.42857143 0.44285714 0.45714286 0.47142857 0.48571429 0.5 0.51428571 0.52857143 0.54285714 0.55714286 0.57142857 0.58571429 0.6 0.61428571 0.62857143 0.64285714 0.65714286 0.67142857 0.68571429 0.7 0.71428571 0.72857143 0.74285714 0.75714286 0.77142857 0.78571429 0.8 0.81428571 0.82857143 0.84285714 0.85714286 0.87142857 0.88571429 0.9 0.91428571 0.92857143 0.94285714 0.95714286 0.97142857 0.98571429 1 1 1 1 1 1
  arc A58 (-4.8994, 5.2759) -> (-5.2759, 4.8994) centre (0, 0) ccw
  spline S29 degree 5 poles (-5.2759, 4.8994) (-5.275, 4.8956) (-5.2731, 4.8878) (-5.2702, 4.8762) (-5.2663, 4.8608) (-5.2613, 4.8416) (-5.2563, 4.8224) (-5.2511, 4.8033) (-5.2459, 4.7843) (-5.2405, 4.7653) (-5.2351, 4.7464) (-5.2296, 4.7275) (-5.224, 4.7087) (-5.2183, 4.69) (-5.2126, 4.6714) (-5.2067, 4.6528) (-5.2007, 4.6343) (-5.1947, 4.6158) (-5.1886, 4.5975) (-5.1823, 4.5792) (-5.176, 4.5609) (-5.1696, 4.5428) (-5.1631, 4.5247) (-5.1565, 4.5067) (-5.1498, 4.4887) (-5.1431, 4.4709) (-5.1362, 4.4531) (-5.1292, 4.4354) (-5.1222, 4.4177) (-5.115, 4.4002) (-5.1078, 4.3827) (-5.1004, 4.3653) (-5.093, 4.348) (-5.0855, 4.3308) (-5.0779, 4.3137) (-5.0701, 4.2966) (-5.0623, 4.2796) (-5.0544, 4.2628) (-5.0464, 4.246) (-5.0383, 4.2293) (-5.0301, 4.2126) (-5.0218, 4.1961) (-5.0134, 4.1797) (-5.0049, 4.1634) (-4.9963, 4.1472) (-4.9876, 4.131) (-4.9788, 4.115) (-4.9698, 4.0991) (-4.9608, 4.0832) (-4.9517, 4.0675) (-4.9425, 4.0519) (-4.9331, 4.0364) (-4.9236, 4.0211) (-4.914, 4.0058) (-4.9043, 3.9907) (-4.8945, 3.9757) (-4.8846, 3.9608) (-4.8746, 3.946) (-4.8644, 3.9313) (-4.8542, 3.9168) (-4.8438, 3.9024) (-4.8332, 3.8883) (-4.8224, 3.8743) (-4.8115, 3.8605) (-4.8004, 3.8469) (-4.7892, 3.8334) (-4.7779, 3.82) (-4.7665, 3.8068) (-4.755, 3.7937) (-4.7433, 3.7808) (-4.7312, 3.7684) (-4.7211, 3.7589) (-4.7133, 3.7521) (-4.708, 3.7477) (-4.7053, 3.7456) knots -1 -1 -1 -1 -1 -1 -0.98571429 -0.97142857 -0.95714286 -0.94285714 -0.92857143 -0.91428571 -0.9 -0.88571429 -0.87142857 -0.85714286 -0.84285714 -0.82857143 -0.81428571 -0.8 -0.78571429 -0.77142857 -0.75714286 -0.74285714 -0.72857143 -0.71428571 -0.7 -0.68571429 -0.67142857 -0.65714286 -0.64285714 -0.62857143 -0.61428571 -0.6 -0.58571429 -0.57142857 -0.55714286 -0.54285714 -0.52857143 -0.51428571 -0.5 -0.48571429 -0.47142857 -0.45714286 -0.44285714 -0.42857143 -0.41428571 -0.4 -0.38571429 -0.37142857 -0.35714286 -0.34285714 -0.32857143 -0.31428571 -0.3 -0.28571429 -0.27142857 -0.25714286 -0.24285714 -0.22857143 -0.21428571 -0.2 -0.18571429 -0.17142857 -0.15714286 -0.14285714 -0.12857143 -0.11428571 -0.1 -0.08571429 -0.07142857 -0.05714286 -0.04285714 -0.02857143 -0.01428571 0 0 0 0 0 0
  line L29 (-4.7053, 3.7456) -> (-4.4368, 3.5318)
  arc A59 (-4.4006, 3.2564) -> (-4.4368, 3.5318) centre (-4.5613, 3.3754) ccw
  arc A60 (-4.4006, 3.2564) -> (-4.6925, 2.8194) centre (0, 0) ccw
  arc A61 (-4.9609, 2.7475) -> (-4.6925, 2.8194) centre (-4.864, 2.9224) ccw
  line L30 (-4.9609, 2.7475) -> (-5.2611, 2.9137)
  spline S30 degree 5 poles (-5.2611, 2.9137) (-5.2641, 2.9154) (-5.2702, 2.9187) (-5.2795, 2.9233) (-5.2921, 2.929) (-5.3082, 2.9354) (-5.3245, 2.9413) (-5.3411, 2.9469) (-5.3577, 2.9523) (-5.3744, 2.9576) (-5.3911, 2.9628) (-5.4079, 2.9679) (-5.4248, 2.9727) (-5.4419, 2.9773) (-5.459, 2.9817) (-5.4763, 2.9858) (-5.4936, 2.9897) (-5.5111, 2.9934) (-5.5286, 2.997) (-5.5461, 3.0005) (-5.5637, 3.0038) (-5.5814, 3.007) (-5.5992, 3.0101) (-5.617, 3.0129) (-5.6349, 3.0156) (-5.6528, 3.0182) (-5.6709, 3.0206) (-5.6889, 3.0229) (-5.7071, 3.025) (-5.7252, 3.027) (-5.7435, 3.0289) (-5.7618, 3.0307) (-5.7801, 3.0323) (-5.7985, 3.0338) (-5.8169, 3.0351) (-5.8354, 3.0363) (-5.8539, 3.0374) (-5.8725, 3.0384) (-5.8911, 3.0392) (-5.9098, 3.04) (-5.9285, 3.0406) (-5.9473, 3.0411) (-5.9661, 3.0414) (-5.9849, 3.0417) (-6.0038, 3.0418) (-6.0227, 3.0418) (-6.0416, 3.0417) (-6.0606, 3.0414) (-6.0796, 3.0411) (-6.0987, 3.0406) (-6.1178, 3.0401) (-6.1369, 3.0394) (-6.1561, 3.0386) (-6.1753, 3.0377) (-6.1945, 3.0366) (-6.2138, 3.0355) (-6.2331, 3.0342) (-6.2524, 3.0329) (-6.2718, 3.0314) (-6.2911, 3.0298) (-6.3105, 3.0281) (-6.33, 3.0263) (-6.3495, 3.0244) (-6.3689, 3.0224) (-6.3885, 3.0203) (-6.408, 3.018) (-6.4276, 3.0157) (-6.4472, 3.0133) (-6.4668, 3.0107) (-6.4864, 3.008) (-6.5061, 3.0053) (-6.5219, 3.003) (-6.5337, 3.0012) (-6.5416, 3) (-6.5455, 2.9994) knots 0 0 0 0 0 0 0.01428571 0.02857143 0.04285714 0.05714286 0.07142857 0.08571429 0.1 0.11428571 0.12857143 0.14285714 0.15714286 0.17142857 0.18571429 0.2 0.21428571 0.22857143 0.24285714 0.25714286 0.27142857 0.28571429 0.3 0.31428571 0.32857143 0.34285714 0.35714286 0.37142857 0.38571429 0.4 0.41428571 0.42857143 0.44285714 0.45714286 0.47142857 0.48571429 0.5 0.51428571 0.52857143 0.54285714 0.55714286 0.57142857 0.58571429 0.6 0.61428571 0.62857143 0.64285714 0.65714286 0.67142857 0.68571429 0.7 0.71428571 0.72857143 0.74285714 0.75714286 0.77142857 0.78571429 0.8 0.81428571 0.82857143 0.84285714 0.85714286 0.87142857 0.88571429 0.9 0.91428571 0.92857143 0.94285714 0.95714286 0.97142857 0.98571429 1 1 1 1 1 1
  arc A62 (-6.5455, 2.9994) -> (-6.7493, 2.5075) centre (0, 0) ccw
  spline S31 degree 5 poles (-6.7493, 2.5075) (-6.7469, 2.5043) (-6.7422, 2.4978) (-6.7351, 2.4882) (-6.7256, 2.4755) (-6.7136, 2.4596) (-6.7016, 2.4438) (-6.6895, 2.4282) (-6.6774, 2.4126) (-6.6652, 2.3971) (-6.653, 2.3817) (-6.6407, 2.3664) (-6.6283, 2.3512) (-6.6159, 2.336) (-6.6034, 2.321) (-6.5909, 2.3061) (-6.5783, 2.2913) (-6.5657, 2.2766) (-6.553, 2.2619) (-6.5402, 2.2474) (-6.5274, 2.233) (-6.5145, 2.2186) (-6.5016, 2.2044) (-6.4886, 2.1903) (-6.4756, 2.1763) (-6.4625, 2.1624) (-6.4493, 2.1486) (-6.4361, 2.1349) (-6.4229, 2.1213) (-6.4095, 2.1078) (-6.3962, 2.0944) (-6.3827, 2.0812) (-6.3692, 2.068) (-6.3557, 2.055) (-6.3421, 2.0421) (-6.3284, 2.0293) (-6.3147, 2.0166) (-6.301, 2.004) (-6.2871, 1.9916) (-6.2733, 1.9792) (-6.2593, 1.967) (-6.2453, 1.955) (-6.2313, 1.943) (-6.2172, 1.9312) (-6.203, 1.9195) (-6.1888, 1.9079) (-6.1745, 1.8965) (-6.1602, 1.8852) (-6.1458, 1.874) (-6.1313, 1.863) (-6.1168, 1.8521) (-6.1023, 1.8414) (-6.0876, 1.8308) (-6.0729, 1.8204) (-6.0582, 1.8101) (-6.0434, 1.8) (-6.0285, 1.79) (-6.0136, 1.7802) (-5.9986, 1.7705) (-5.9836, 1.761) (-5.9685, 1.7518) (-5.9533, 1.7427) (-5.938, 1.7339) (-5.9226, 1.7254) (-5.9071, 1.717) (-5.8916, 1.7089) (-5.8761, 1.7008) (-5.8605, 1.6929) (-5.8448, 1.6852) (-5.8291, 1.6778) (-5.8132, 1.671) (-5.8002, 1.6661) (-5.7904, 1.6628) (-5.7838, 1.6608) (-5.7805, 1.6598) knots -1 -1 -1 -1 -1 -1 -0.98571429 -0.97142857 -0.95714286 -0.94285714 -0.92857143 -0.91428571 -0.9 -0.88571429 -0.87142857 -0.85714286 -0.84285714 -0.82857143 -0.81428571 -0.8 -0.78571429 -0.77142857 -0.75714286 -0.74285714 -0.72857143 -0.71428571 -0.7 -0.68571429 -0.67142857 -0.65714286 -0.64285714 -0.62857143 -0.61428571 -0.6 -0.58571429 -0.57142857 -0.55714286 -0.54285714 -0.52857143 -0.51428571 -0.5 -0.48571429 -0.47142857 -0.45714286 -0.44285714 -0.42857143 -0.41428571 -0.4 -0.38571429 -0.37142857 -0.35714286 -0.34285714 -0.32857143 -0.31428571 -0.3 -0.28571429 -0.27142857 -0.25714286 -0.24285714 -0.22857143 -0.21428571 -0.2 -0.18571429 -0.17142857 -0.15714286 -0.14285714 -0.12857143 -0.11428571 -0.1 -0.08571429 -0.07142857 -0.05714286 -0.04285714 -0.02857143 -0.01428571 0 0 0 0 0 0
  line L31 (-5.7805, 1.6598) -> (-5.4506, 1.5651)
  arc A63 (-5.3118, 1.3245) -> (-5.4506, 1.5651) centre (-5.5058, 1.3729) ccw
  circle A64 centre (0, 0) radius 0.9
  circle A65 centre (0, 0) radius 2.55
  dimension "d9" = 5.1
  constraint concentric A0 A65
  measures "d9" diameter of A65
extrude "Extrude3" cut sketch "Sketch4" against normal blind 1 contours A65 bodies 1
sketch "Sketch5" plane through (0, 0, 0) normal (0, 0, 1) x (1, 0, 0)
  circle A0 centre (0, 0) radius 2.55
  dimension "d12" = 5.1
  constraint coincident A0.centre origin
  measures "d12" diameter of A0
extrude "Extrude4" cut sketch "Sketch5" along normal blind 2 bodies 1
sketch "Sketch6" plane through (0, 0, 0) normal (0, 0, 1) x (1, 0, 0)
  circle A0 centre (0, 0) radius 0.95
  dimension "d15" = 1.9
  constraint coincident A0.centre origin
  measures "d15" diameter of A0
sketch "Sketch7" plane through (0, 0, 3) normal (0, 0, 1) x (-1, 0, 0)
  circle A0 centre (0, 0) radius 0.9
  circle A1 centre (0, 0) radius 2.55
  circle A2 centre (0, 0) radius 0.95
  dimension "d16" = 1.9
  constraint concentric A0 A2
  measures "d16" diameter of A2
extrude "Extrude5" cut sketch "Sketch7" against normal blind 1 contours A2 bodies 1